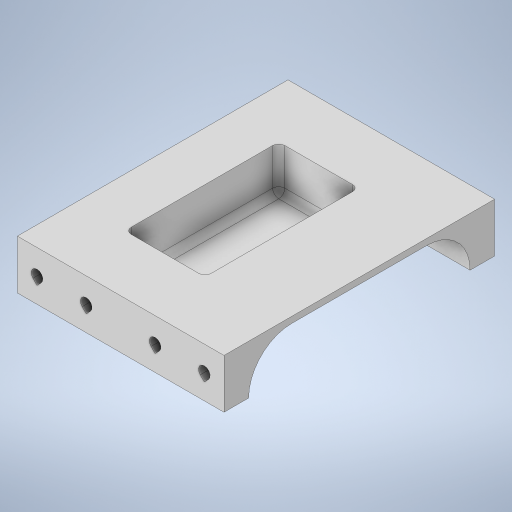
# Autodesk Inventor part: hub
Saved by Autodesk Inventor 2024 (Build 280153000, 153)
## iProperties
Created: 2023-11-29
Part Number: hub
Material: Generic
Document SubType Name: Modeling
Designer: CJ110
Density: 1 g/cm^3
Appearance: Default
Author: CJ110
## iProperties of the stored document hub_3DPrint.ipt
Created: 2023-11-30
Part Number: hub_3DPrint
Material: Generic
Document SubType Name: Modeling
Designer: CJ110
Density: 1 g/cm^3
Appearance: Default
Author: CJ110
Autodesk Inventor part; units mm, degrees
ref_plane "YZ Plane" through (0, 0, 0) normal (1, 0, 0) x (0, 1, 0)
ref_plane "XZ Plane" through (0, 0, 0) normal (0, 1, 0) x (-1, 0, 0)
ref_plane "XY Plane" through (0, 0, 0) normal (0, 0, 1) x (1, 0, 0)
sketch "Sketch1" plane through (0, 0, 0) normal (0, 1, 0) x (-1, 0, 0)
  line L0 (0, 0) -> (106.68, 0)
  line L1 (106.68, 0) -> (106.68, 139.7)
  line L2 (106.68, 139.7) -> (0, 139.7)
  line L3 (0, 139.7) -> (0, 0)
  dimension "d0" = 139.7
  dimension "d1" = 106.68
  constraints: 8 end point, 2 parallel, 1 horizontal, 1 perpendicular
  measures "d0" distance of L0.end L1.end
  measures "d1" distance of L1.end L2.end
extrude "Extrusion1" add sketch "Sketch1" along normal blind 25.4
sketch "Sketch2" plane through (0, 25.4, 0) normal (0, 1, 0) x (1, 0, 0)
  line L0 (-81.28, -109.5375) -> (-40.005, -109.5375)
  line L1 (-40.005, -109.5375) -> (-40.005, -30.1625)
  line L2 (-40.005, -30.1625) -> (-81.28, -30.1625)
  line L3 (-81.28, -30.1625) -> (-81.28, -109.5375)
  line L4 (-106.68, -139.7) -> (0, -139.7) projected
  line L5 (-106.68, 0) -> (-106.68, -139.7) projected
  line L6 (-106.68, -139.7) -> (0, -139.7) projected
  line L7 (0, -139.7) -> (0, 0) projected
  line L8 (0, 0) -> (-106.68, 0) projected
  line L9 (-106.68, 0) -> (-106.68, -139.7) projected
  line L10 (-106.68, -69.85) -> (0, -69.85) construction
  point P0 (-81.28, -69.85)
  dimension "d4" = 41.275
  dimension "d5" = 79.375
  dimension "d6" = 25.4
  constraints: 10 end point, 3 midpoint, 2 parallel, 1 horizontal, 1 perpendicular, 1 point on line
  measures "d4" distance between parallel lines of L1 L3
  measures "d5" distance between parallel lines of L2 L0
  measures "d6" distance between parallel lines of L3 L5
extrude "Extrusion2" cut sketch "Sketch2" against normal blind 22.225 contours L3 L2 L1 L0
ref_plane "Work Plane1" through (-106.68, 0, 69.85) normal (0, 0, 1) x (1, 0, 0)
ref_plane "Work Plane2" through (-53.34, 0, 139.7) normal (1, 0, 0) x (0, 0, -1)
sketch "Sketch3" plane through (0, 25.4, 0) normal (0, 1, 0) x (1, 0, 0)
  circle A0 centre (-100.33, -142.24) radius 1.27
  line L0 (-106.68, 0) -> (-106.68, -139.7) projected
  line L1 (-106.68, -69.85) -> (0, -69.85) construction
  line L2 (0, -139.7) -> (0, 0) projected
  line L3 (-81.28, -30.1625) -> (-40.005, -30.1625) projected
  line L4 (-40.005, -30.1625) -> (-40.005, -109.5375) projected
  line L5 (-40.005, -109.5375) -> (-81.28, -109.5375) projected
  line L6 (-81.28, -109.5375) -> (-81.28, -30.1625) projected
  line L7 (-106.68, 0) -> (-106.68, -139.7) projected
  line L8 (-106.68, -139.7) -> (0, -139.7) projected
  line L9 (0, -139.7) -> (0, 0) projected
  line L10 (0, 0) -> (-106.68, 0) projected
  arc A1 (-104.14, -142.24) -> (-96.52, -142.24) centre (-100.33, -142.24) ccw
  line L11 (-96.52, -142.24) -> (-96.52, -139.7)
  line L12 (-104.14, -139.7) -> (-104.14, -142.24)
  dimension "d9" = 2.54
  dimension "d10" = 7.62
  dimension "d11" = 2.54
  dimension "d16" = 2.54
  constraints: 6 end point, 2 centre point, 2 midpoint, 2 point on circle, 2 point on line, 2 tangent, 1 coincident, 1 perpendicular, 1 vertical
  measures "d9" diameter of A0
  measures "d10" diameter of A1
  measures "d11" distance from line of L8 A0.centre
  measures "d16" distance between parallel lines of L0 L12
extrude "Extrusion3" [suppressed]
mirror "Mirror2" [suppressed]
fillet "Fillet1" radius 3.175 8 edges at (-81.28, 3.175, 69.85) (-60.6425, 3.175, 30.1625) (-40.005, 3.175, 69.85) (-60.6425, 3.175, 109.5375) (-40.005, 14.2875, 109.5375) (-81.28, 14.2875, 109.5375) (-40.005, 14.2875, 30.1625) (-81.28, 14.2875, 30.1625)
sketch "Sketch4" plane through (-106.68, 0, 139.7) normal (0, 0, 1) x (1, 0, 0)
  line L0 (0, 25.4) -> (106.68, 25.4) projected
  line L1 (0, 0) -> (0, 25.4) projected
  line L2 (0, 0) -> (106.68, 0) projected
  line L3 (106.68, 0) -> (106.68, 25.4) projected
  circle A0 centre (96.52, 12.7) radius 3
  circle A1 centre (71.12, 12.7) radius 3
  line L4 (106.68, 12.7) -> (0, 12.7) construction
  point P0 (106.68, 0)
  dimension "d17" = 6
  dimension "d18" = 10.16
  dimension "d22" = 25.4
  constraints: 2 centre point, 2 end point, 2 midpoint, 2 point on line, 1 equal radius
  measures "d17" diameter of A0
  measures "d18" distance from line of L3 A0.centre
  measures "d22" distance of A0.centre A1.centre
extrude "Extrusion4" cut sketch "Sketch4" against normal blind 11 contours A0 | A1
mirror "Mirror3" about plane through (-106.68, 0, 69.85) normal (0, 0, 1) of "Extrusion4"
mirror "Mirror4" about plane through (-53.34, 0, 139.7) normal (1, 0, 0) of "Extrusion4", "Mirror3"
sketch "Sketch6" plane through (0, 0, 139.7) normal (1, 0, 0) x (0, 0, -1)
  line L0 (0, 0) -> (139.7, 0) projected
  line L1 (139.7, 0) -> (139.7, 25.4) projected
  line L2 (0, 25.4) -> (139.7, 25.4) projected
  line L3 (0, 0) -> (0, 25.4) projected
  line L4 (12.7, 0) -> (127, 0)
  line L5 (127, 0) -> (127, 22.225)
  line L6 (127, 22.225) -> (12.7, 22.225)
  line L7 (12.7, 22.225) -> (12.7, 0)
  arc A0 (34.925, 22.225) -> (12.7, 0) centre (34.925, 0) ccw
  arc A1 (127, 0) -> (104.775, 22.225) centre (104.775, 0) ccw
  point P0 (127, 0)
  dimension "d23" = 3.175
  dimension "d24" = 12.7
  dimension "d25" = 12.7
  constraints: 8 end point, 4 point on circle, 4 tangent, 3 point on line, 2 centre point, 2 parallel, 1 horizontal, 1 perpendicular
  measures "d23" distance between parallel lines of L2 L6
  measures "d24" distance between parallel lines of L3 L7
  measures "d25" distance between parallel lines of L1 L5
extrude "Extrusion5" cut sketch "Sketch6" against normal blind 36.83 contours A0 L6 A1 L0
fillet "Fillet2" radius 6.35 4 edges at (-36.83, 15.7154, 19.2096) (-36.83, 15.7154, 120.4904) (-36.83, 22.225, 69.85) (-36.83, 0, 69.85)
sketch "Sketch7" plane through (-106.68, 0, 0) normal (-1, 0, 0) x (0, 0, 1)
  line L0 (0, 0) -> (139.7, 0) projected
  line L1 (139.7, 0) -> (139.7, 25.4) projected
  line L2 (0, 25.4) -> (139.7, 25.4) projected
  line L3 (0, 0) -> (0, 25.4) projected
  line L4 (12.7, 0) -> (127, 0)
  line L5 (127, 0) -> (127, 22.225)
  line L6 (127, 22.225) -> (12.7, 22.225)
  line L7 (12.7, 22.225) -> (12.7, 0)
  arc A0 (34.925, 22.225) -> (12.7, 0) centre (34.925, 0) ccw
  arc A1 (127, 0) -> (104.775, 22.225) centre (104.775, 0) ccw
  point P0 (0, 0)
  dimension "d29" = 3.175
  dimension "d30" = 12.7
  dimension "d31" = 12.7
  constraints: 8 end point, 4 point on circle, 4 tangent, 3 point on line, 2 centre point, 2 parallel, 1 horizontal, 1 perpendicular
  measures "d29" distance between parallel lines of L2 L6
  measures "d30" distance between parallel lines of L3 L7
  measures "d31" distance between parallel lines of L1 L5
extrude "Extrusion6" cut sketch "Sketch7" against normal blind 22.225 contours A0 L6 A1 L0
fillet "Fillet3" radius 6.35 4 edges at (-84.455, 0, 69.85) (-84.455, 15.7154, 120.4904) (-84.455, 15.7154, 19.2096) (-84.455, 22.225, 69.85)
sketch "Sketch8" plane through (-106.68, 0, 139.7) normal (0, 0, 1) x (1, 0, 0)
  circle A0 centre (10.16, 12.7) radius 3 projected
  circle A1 centre (35.56, 12.7) radius 3 projected
  circle A2 centre (96.52, 12.7) radius 3 projected
  circle A3 centre (71.12, 12.7) radius 3 projected
  line L0 (0, 0) -> (106.68, 0) projected
  line L1 (106.68, 0) -> (106.68, 25.4) projected
  line L2 (0, 25.4) -> (106.68, 25.4) projected
  line L3 (0, 0) -> (0, 25.4) projected
  line L4 (10.16, 12.7) -> (10.16, 8.4574) construction
  line L5 (35.56, 12.7) -> (35.56, 8.4574) construction
  line L6 (71.12, 12.7) -> (71.12, 8.4574) construction
  line L7 (96.52, 12.7) -> (96.52, 8.4574) construction
  line L8 (71.12, 8.4574) -> (73.2413, 10.5787)
  line L9 (71.12, 8.4574) -> (68.9987, 10.5787)
  line L10 (96.52, 8.4574) -> (98.6413, 10.5787)
  line L11 (96.52, 8.4574) -> (94.3987, 10.5787)
  line L12 (35.56, 8.4574) -> (37.6813, 10.5787)
  line L13 (35.56, 8.4574) -> (33.4387, 10.5787)
  line L14 (10.16, 8.4574) -> (12.2813, 10.5787)
  line L15 (10.16, 8.4574) -> (8.0387, 10.5787)
  circle A4 centre (35.56, 12.7) radius 3 projected
  circle A5 centre (10.16, 12.7) radius 3 projected
  circle A6 centre (96.52, 12.7) radius 3 projected
  point P0 (106.68, 0)
  constraints: 24 end point, 9 tangent, 8 point on circle, 6 perpendicular, 4 vertical
extrude "Extrusion7" cut sketch "Sketch8" against normal up to surface (11 mm away) contours A0 L14 L15 | A1 L12 L13 | A2 L10 L11 | A3 L8 L9
mirror "Mirror5" about plane through (-106.68, 0, 69.85) normal (0, 0, 1) of "Extrusion7"
equation "\"d25\" = d24"
equation "\"d31\" = d30"
body "Solid1"
